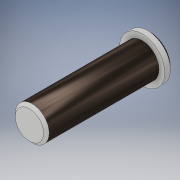
# Autodesk Inventor part: reverse gear crankrod pin 1
Saved by Autodesk Inventor 2017 (Build 210142000, 142)
## iProperties
Created: 2018-10-30
Part Number: reverse gear crankrod pin 1
Material: Generic
Document SubType Name: Modeling
Designer: User
Density: 1 g/cm^3
Appearance: Default
Author: User
Autodesk Inventor part; units mm, degrees
ref_plane "YZ Plane" through (0, 0, 0) normal (1, 0, 0) x (0, 1, 0)
ref_plane "XZ Plane" through (0, 0, 0) normal (0, 1, 0) x (-1, 0, 0)
ref_plane "XY Plane" through (0, 0, 0) normal (0, 0, 1) x (1, 0, 0)
sketch "Sketch1" plane through (0, 0, 0) normal (0, 1, 0) x (-1, 0, 0)
  circle A0 centre (0, 0) radius 4
  dimension "d0" = 8
  constraints: 1 centre point, 1 coincident
  measures "d0" diameter of A0
extrude "Extrusion1" add sketch "Sketch1" along normal blind 1.5
sketch "Sketch2" plane through (0, 0, 0) normal (0, -1, 0) x (1, 0, 0)
  circle A0 centre (0, 0) radius 3
  dimension "d4" = 6
  constraints: 1 centre point, 1 coincident
  measures "d4" diameter of A0
extrude "Extrusion2" add sketch "Sketch2" along normal blind 20
chamfer "Chamfer1" distance 0.5 angle 45 1 edges at (4, 1.5, 0)
chamfer "Chamfer2" distance 0.5 angle 45 1 edges at (-3, -20, 0)
body "Solid1"
